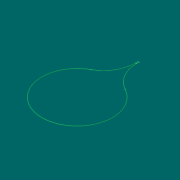
# Autodesk Inventor part: Fiber Loop
Saved by Autodesk Inventor 2016 (Build 200138000, 138)
## iProperties
Created: 2015-08-17
Part Number: Fiber Loop
Material: Glass
Document SubType Name: Modeling
Designer: Cosmic
Density: 2.18 g/cm^3
Appearance: Clear - Green 1
Author: Cosmic
Autodesk Inventor part; units mm, degrees
ref_plane "YZ Plane" through (0, 0, 0) normal (1, 0, 0) x (0, 1, 0)
ref_plane "XZ Plane" through (0, 0, 0) normal (0, 1, 0) x (-1, 0, 0)
ref_plane "XY Plane" through (0, 0, 0) normal (0, 0, 1) x (1, 0, 0)
sketch "Sketch1" plane through (0, 0, 0) normal (0, 0, 1) x (1, 0, 0)
  arc A0 (23.923278, 43.335053) -> (-23.923278, 43.335053) centre (0, 0) ccw
  arc A1 (-23.995772, 43.466371) -> (-26.306921, 42.107819) centre (0, 0) ccw
  arc A2 (-30.316871, 40.574744) -> (-30.724109, 40.267253) centre (0, 0) ccw
  arc A3 (-30.796514, 40.400677) -> (-31.176261, 40.108363) centre (0, 0) ccw
  arc A4 (-1.3, 83.868647) -> (-91.3, 83.868647) centre (-46.3, 83.868647) ccw
  arc A5 (-1.15, 83.868647) -> (-91.45, 83.868647) centre (-46.3, 83.868647) ccw
  arc A6 (-23.995772, 43.466371) -> (-18.180674, 47.274577) centre (-46.3, 83.868647) ccw
  arc A7 (-26.306921, 42.107819) -> (-23.923278, 43.335053) centre (-46.3, 83.868647) ccw
  arc A8 (24.551566, 44.473145) -> (91.3, 83.868647) centre (46.3, 83.868647) ccw
  arc A9 (22.173978, 45.705084) -> (24.479071, 44.341827) centre (46.3, 83.868647) ccw
  arc A10 (17.777802, 47.587706) -> (18.180674, 47.274577) centre (46.3, 83.868647) ccw
  arc A11 (17.328095, 47.753294) -> (17.703477, 47.455341) centre (46.3, 83.868647) ccw
  line L0 (-46.3, 83.868647) -> (46.3, 83.868647)
  arc A12 (-26.860934, 43.117632) -> (-30.796514, 40.400677) centre (0, 0) ccw
  arc A13 (-24.479071, 44.341827) -> (-30.316871, 40.574744) centre (0, 0) ccw
  arc A14 (-30.316871, 40.574744) -> (-23.995772, 43.466371) centre (-46.3, 83.868647) ccw
  arc A15 (-30.724109, 40.267253) -> (-26.306921, 42.107819) centre (-46.3, 83.868647) ccw
  arc A16 (-30.796514, 40.400677) -> (-30.316871, 40.574744) centre (-46.3, 83.868647) ccw
  arc A17 (-30.724109, 40.267253) -> (30.724109, 40.267253) centre (0, 0) ccw
  arc A18 (-0.15, 83.868647) -> (-92.45, 83.868647) centre (-46.3, 83.868647) ccw
  arc A19 (-31.176261, 40.108363) -> (31.176261, 40.108363) centre (0, 0) ccw
  arc A20 (30.724109, 40.267253) -> (30.316871, 40.574744) centre (0, 0) ccw
  arc A21 (31.176261, 40.108363) -> (30.796514, 40.400677) centre (0, 0) ccw
  arc A22 (-92.45, 83.868647) -> (-30.796514, 40.400677) centre (-46.3, 83.868647) ccw
  arc A23 (-31.176261, 40.108363) -> (-30.724109, 40.267253) centre (-46.3, 83.868647) ccw
  arc A24 (0, 83.868647) -> (-92.6, 83.868647) centre (-46.3, 83.868647) ccw
  arc A25 (-18.180674, 47.274577) -> (-17.777802, 47.587706) centre (-46.3, 83.868647) ccw
  arc A26 (-17.777802, 47.587706) -> (-22.173978, 45.705084) centre (0, 0) ccw
  arc A27 (-17.777802, 47.587706) -> (-0.15, 83.868647) centre (-46.3, 83.868647) ccw
  arc A28 (-24.551566, 44.473145) -> (-1.3, 83.868647) centre (-46.3, 83.868647) ccw
  arc A29 (-22.173978, 45.705084) -> (-1.15, 83.868647) centre (-46.3, 83.868647) ccw
  arc A30 (-17.328095, 47.753294) -> (0, 83.868647) centre (-46.3, 83.868647) ccw
  arc A31 (-21.614664, 44.698197) -> (-23.995772, 43.466371) centre (0, 0) ccw
  arc A32 (-23.923278, 43.335053) -> (23.923278, 43.335053) centre (0, 0) ccw
  arc A33 (-26.860934, 43.117632) -> (-24.479071, 44.341827) centre (-46.3, 83.868647) ccw
  arc A34 (-91.45, 83.868647) -> (-26.860934, 43.117632) centre (-46.3, 83.868647) ccw
  arc A35 (-26.306921, 42.107819) -> (26.306921, 42.107819) centre (0, 0) ccw
  arc A36 (-91.3, 83.868647) -> (-24.551566, 44.473145) centre (-46.3, 83.868647) ccw
  arc A37 (-92.6, 83.868647) -> (-31.176261, 40.108363) centre (-46.3, 83.868647) ccw
  arc A38 (26.306921, 42.107819) -> (23.995772, 43.466371) centre (0, 0) ccw
  arc A39 (-24.551566, 44.473145) -> (-26.860934, 43.117632) centre (0, 0) ccw
  arc A40 (-24.479071, 44.341827) -> (-22.173978, 45.705084) centre (-46.3, 83.868647) ccw
  arc A41 (-23.923278, 43.335053) -> (-21.614664, 44.698197) centre (-46.3, 83.868647) ccw
  arc A42 (-21.614664, 44.698197) -> (-17.703477, 47.455341) centre (-46.3, 83.868647) ccw
  arc A43 (-22.173978, 45.705084) -> (-24.551566, 44.473145) centre (0, 0) ccw
  arc A44 (-18.180674, 47.274577) -> (-24.479071, 44.341827) centre (0, 0) ccw
  arc A45 (21.614664, 44.698197) -> (-21.614664, 44.698197) centre (0, 0) ccw
  arc A46 (-17.703477, 47.455341) -> (-17.328095, 47.753294) centre (-46.3, 83.868647) ccw
  arc A47 (-17.328095, 47.753294) -> (-17.777802, 47.587706) centre (0, 0) ccw
  arc A48 (17.328095, 47.753294) -> (-17.328095, 47.753294) centre (0, 0) ccw
  arc A49 (-17.703477, 47.455341) -> (-18.180674, 47.274577) centre (0, 0) ccw
  arc A50 (17.703477, 47.455341) -> (-17.703477, 47.455341) centre (0, 0) ccw
  arc A51 (1.15, 83.868647) -> (22.173978, 45.705084) centre (46.3, 83.868647) ccw
  arc A52 (1.3, 83.868647) -> (24.551566, 44.473145) centre (46.3, 83.868647) ccw
  arc A53 (0, 83.868647) -> (17.328095, 47.753294) centre (46.3, 83.868647) ccw
  arc A54 (0.15, 83.868647) -> (17.777802, 47.587706) centre (46.3, 83.868647) ccw
  arc A55 (17.703477, 47.455341) -> (21.614664, 44.698197) centre (46.3, 83.868647) ccw
  arc A56 (17.777802, 47.587706) -> (17.328095, 47.753294) centre (0, 0) ccw
  arc A57 (18.180674, 47.274577) -> (23.995772, 43.466371) centre (46.3, 83.868647) ccw
  arc A58 (21.614664, 44.698197) -> (23.923278, 43.335053) centre (46.3, 83.868647) ccw
  arc A59 (22.173978, 45.705084) -> (17.777802, 47.587706) centre (0, 0) ccw
  arc A60 (23.995772, 43.466371) -> (30.316871, 40.574744) centre (46.3, 83.868647) ccw
  arc A61 (18.180674, 47.274577) -> (17.703477, 47.455341) centre (0, 0) ccw
  arc A62 (24.479071, 44.341827) -> (18.180674, 47.274577) centre (0, 0) ccw
  arc A63 (24.479071, 44.341827) -> (26.860934, 43.117632) centre (46.3, 83.868647) ccw
  arc A64 (24.551566, 44.473145) -> (22.173978, 45.705084) centre (0, 0) ccw
  arc A65 (23.923278, 43.335053) -> (26.306921, 42.107819) centre (46.3, 83.868647) ccw
  arc A66 (23.995772, 43.466371) -> (21.614664, 44.698197) centre (0, 0) ccw
  arc A67 (26.306921, 42.107819) -> (30.724109, 40.267253) centre (46.3, 83.868647) ccw
  arc A68 (30.316871, 40.574744) -> (30.796514, 40.400677) centre (46.3, 83.868647) ccw
  arc A69 (91.3, 83.868647) -> (1.3, 83.868647) centre (46.3, 83.868647) ccw
  arc A70 (26.860934, 43.117632) -> (91.45, 83.868647) centre (46.3, 83.868647) ccw
  arc A71 (30.316871, 40.574744) -> (24.479071, 44.341827) centre (0, 0) ccw
  arc A72 (26.860934, 43.117632) -> (24.551566, 44.473145) centre (0, 0) ccw
  arc A73 (30.796514, 40.400677) -> (26.860934, 43.117632) centre (0, 0) ccw
  arc A74 (91.45, 83.868647) -> (1.15, 83.868647) centre (46.3, 83.868647) ccw
  arc A75 (30.724109, 40.267253) -> (31.176261, 40.108363) centre (46.3, 83.868647) ccw
  arc A76 (31.176261, 40.108363) -> (92.6, 83.868647) centre (46.3, 83.868647) ccw
  arc A77 (30.796514, 40.400677) -> (92.45, 83.868647) centre (46.3, 83.868647) ccw
  arc A78 (92.45, 83.868647) -> (0.15, 83.868647) centre (46.3, 83.868647) ccw
  arc A79 (92.6, 83.868647) -> (0, 83.868647) centre (46.3, 83.868647) ccw
  dimension "d16" = 0.15
  dimension "d17" = 1
  dimension "d18" = 0.15
  dimension "d19" = 99
  dimension "d20" = 0.15
  dimension "d21" = 1
  dimension "d22" = 0.15
  dimension "d23" = 90
  dimension "d28" = 0.15
  dimension "d29" = 1
  dimension "d30" = 0.15
  dimension "d31" = 90
  constraints: 181 point on circle, 80 centre point, 10 coincident, 3 tangent, 19 other
  measures "d16" radial gap between concentric circles of A1 A0
  measures "d17" radial gap between concentric circles of A2 A1
  measures "d18" radial gap between concentric circles of A3 A2
  measures "d19" diameter of A0
  measures "d20" radial gap between concentric circles of A5 A4
  measures "d21" radial gap between concentric circles of A6 A5
  measures "d22" radial gap between concentric circles of A7 A6
  measures "d23" diameter of A4
  measures "d28" radial gap between concentric circles of A9 A8
  measures "d29" radial gap between concentric circles of A10 A9
  measures "d30" radial gap between concentric circles of A11 A10
  measures "d31" diameter of A8
sketch "Sketch1 outline for Extrusion1" plane through (0, 0, 0) normal (0, 0, 1) x (1, 0, 0)
  arc A0 (-24.479071, 44.341827) -> (24.479071, 44.341827) centre (0, 0) ccw
  arc A1 (24.479071, 44.341827) -> (1.15, 83.868647) centre (46.3, 83.868647) cw
  line L0 (1.15, 83.868647) -> (0.15, 83.868647)
  arc A2 (0.15, 83.868647) -> (23.995772, 43.466371) centre (46.3, 83.868647) ccw
  arc A3 (23.995772, 43.466371) -> (-23.995772, 43.466371) centre (0, 0) cw
  arc A4 (-23.995772, 43.466371) -> (-0.15, 83.868647) centre (-46.3, 83.868647) ccw
  line L1 (-0.15, 83.868647) -> (-1.15, 83.868647)
  arc A5 (-1.15, 83.868647) -> (-24.479071, 44.341827) centre (-46.3, 83.868647) cw
extrude "Extrusion1" add sketch "Sketch1 outline for Extrusion1" along normal blind 1
fillet "Fillet1" radius 0.5 12 edges at (-25.1605, 42.8027, 1) (6.5561, 60.4114, 1) (-6.5561, 60.4114, 1) (-3.7284, -50.5126, 1) (7.4172, 60.9197, 1) (-7.4172, 60.9197, 1) (-3.7284, -50.5126, 0) (-7.4172, 60.9197, 0) (7.4172, 60.9197, 0) (-25.1605, 42.8027, 0) (6.5561, 60.4114, 0) (-6.5561, 60.4114, 0)
sketch "Sketch2" plane through (0.65, 83.868647, 0.5) normal (0, 1, 0) x (1, 0, 0)
  circle A0 centre (0, 0) radius 0.5 projected
  circle A1 centre (-1.3, 0) radius 0.5 projected
  point P0 (-0.65, 0.5)
extrude "Extrusion2" add sketch "Sketch2" along normal blind 3
equation "\"d16\" = OpticalFiberClearence"
equation "\"d17\" = OpticalFiberDiameter"
equation "\"d18\" = OpticalFiberClearence"
equation "\"d20\" = OpticalFiberClearence"
equation "\"d21\" = OpticalFiberDiameter"
equation "\"d22\" = OpticalFiberClearence"
equation "\"d23\" = LoopSmallTrackDiameter"
equation "\"d28\" = OpticalFiberClearence"
equation "\"d29\" = OpticalFiberDiameter"
equation "\"d30\" = OpticalFiberClearence"
equation "\"d31\" = LoopSmallTrackDiameter"
equation "\"d36\" = OpticalFiberDiameter"
equation "\"d38\" = 0.5 * OpticalFiberDiameter"
equation "\"d39\" = ScintillatorEdgeClearence - MPPCDepth"
equation "\"OpticalFiberDiameter\" = 1"
equation "\"OpticalFiberClearence\" = 0.15"
equation "\"ScintillatorEdgeClearence\" = 3"
equation "\"MPPCDepth\" = 0"
equation "\"LoopLargeTrackRatio\" = 1.1"
equation "\"LoopSmallTrackDiameter\" = 90"
equation "\"d24\" = 0.05"
equation "\"d25\" = 1"
equation "\"d32\" = 0.05"
equation "\"d33\" = 1"
equation "\"FiberSensorClerence\" = 0.5"
equation "\"SmallTrackDiameter\" = 175"
equation "\"ScintillatorWidth\" = 145"
equation "\"ScintillatorHeight\" = 145"
equation "\"ShallowTrackDepth\" = 1.3"
equation "\"MPPCClearence\" = 0.075"
equation "\"MPPCSensorClearence\" = 1.45"
equation "\"MPPCSensorOffsett\" = 2.105"
equation "\"MPPCWidth\" = 5.9"
equation "\"MPPCHeight\" = 6.55"
equation "\"FiberEdgeOffsett\" = 5"
equation "\"LongFiberAngle\" = 30deg"
equation "\"ShortFiberAngle\" = 78deg"
equation "\"MountingScrewDepth\" = 4"
body "Solid1"
